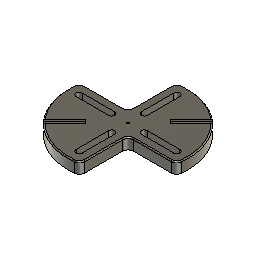
Baseplate (Autodesk Fusion 360 design; units mm, degrees)
part number: 2026-04-13-15-28-07-632
Autodesk Fusion 360 part; units mm, degrees
sketch "Sketch14" plane through (0, 0, 0) normal (0, 0, 1) x (1, 0, 0)
  circle A0 centre (0, 0) radius 55
  dimension "d53" = 110
  constraint coincident A0.centre origin
  measures "d53" diameter of A0
extrude "Extrude9" add sketch "Sketch14" along normal blind 10
sketch "Sketch15" plane through (0, 0, 10) normal (0, 0, 1) x (-1, 0, 0)
  circle A0 centre (0, 0) radius 55
  circle A1 centre (0, 0) radius 15
  circle A2 centre (0, 0) radius 45
  line L0 (-15, 2.8) -> (-45, 2.8)
  arc A3 (-45, 2.8) -> (-45, -2.8) centre (-45, 0) ccw
  line L1 (-45, -2.8) -> (-15, -2.8)
  arc A4 (-15, -2.8) -> (-15, 2.8) centre (-15, 0) ccw
  line L2 (-15, 0) -> (-45, 0) construction
  dimension "d56" = 30
  dimension "d57" = 90
  dimension "d58" = 5.6
  constraint coincident A0.centre A1.centre
  constraint concentric A1 A2
  constraint tangent L0 A3
  constraint tangent A3 L1
  constraint parallel L0 L1
  constraint tangent L1 A4
  constraint tangent L0 A4
  constraint coincident A2 A3.centre
  constraint horizontal L2
  constraint coincident A1 A4.centre
  measures "d56" diameter of A1
  measures "d57" diameter of A2
  measures "d58" diameter of A3
extrude "Extrude10" cut sketch "Sketch15" against normal blind 10 contours A1 A4 | A1 A2 L0 L1 A4 | A2 L0 A3 L1 picked at (-14.0473, 0) picked at (-34.958, -1.556)
pattern_circular "C-Pattern3" count 4 over 360 about axis through (0, 0, 1.75) along (0, 0, 1) of "Extrude10"
sketch "Sketch16" plane through (0, 0, 10) normal (0, 0, 1) x (-1, 0, 0)
  line L0 (2.8, 45) -> (2.8, 15)
  arc A0 (-2.8, 15) -> (2.8, 15) centre (0, 15) ccw
  line L1 (-2.8, 15) -> (-2.8, 45)
  arc A1 (2.8, 45) -> (-2.8, 45) centre (0, 45) ccw
  line L2 (45, -2.8) -> (15, -2.8)
  arc A2 (15, 2.8) -> (15, -2.8) centre (15, 0) ccw
  line L3 (15, 2.8) -> (45, 2.8)
  arc A3 (45, -2.8) -> (45, 2.8) centre (45, 0) ccw
  line L4 (-2.8, -45) -> (-2.8, -15)
  arc A4 (2.8, -15) -> (-2.8, -15) centre (0, -15) ccw
  line L5 (2.8, -15) -> (2.8, -45)
  arc A5 (-2.8, -45) -> (2.8, -45) centre (0, -45) ccw
  line L6 (-45, 2.8) -> (-15, 2.8)
  arc A6 (-15, -2.8) -> (-15, 2.8) centre (-15, 0) ccw
  line L7 (-15, -2.8) -> (-45, -2.8)
  arc A7 (-45, 2.8) -> (-45, -2.8) centre (-45, 0) ccw
  circle A8 centre (0, 0) radius 55
  line L8 (38.3252, 39.4566) -> (-39.4566, -38.3252)
  line L9 (-39.4566, -38.3252) -> (-38.3252, -39.4566)
  line L10 (-38.3252, -39.4566) -> (39.4566, 38.3252)
  line L11 (39.4566, 38.3252) -> (38.3252, 39.4566)
  line L12 (38.3252, 39.4566) -> (-38.3252, -39.4566) construction
  line L13 (-39.4566, -38.3252) -> (39.4566, 38.3252) construction
  line L14 (18.8798, 20.0111) -> (-20.0111, -18.8798)
  line L15 (-20.0111, -18.8798) -> (-18.8798, -20.0111)
  line L16 (-18.8798, -20.0111) -> (20.0111, 18.8798)
  line L17 (20.0111, 18.8798) -> (18.8798, 20.0111)
  line L18 (18.8798, 20.0111) -> (-18.8798, -20.0111) construction
  line L19 (-20.0111, -18.8798) -> (20.0111, 18.8798) construction
  dimension "d63" = 110
  dimension "d64" = 1.6
  dimension "d65" = 55
  dimension "d66" = 1.6
  constraint perpendicular L8 L9
  constraint parallel L8 L10
  constraint parallel L9 L11
  constraint coincident L12 A8.centre
  constraint coincident L13 A8.centre
  constraint coincident A8.centre origin
  constraint perpendicular L14 L15
  constraint parallel L14 L16
  constraint parallel L15 L17
  constraint coincident L18 A8.centre
  constraint coincident L19 A8.centre
  measures "d63" distance of L9.end L10.end
  measures "d64" distance of L8.end L9.end
  measures "d65" distance of L15.end L16.end
  measures "d66" distance of L14.end L15.end
extrude "Extrude11" add sketch "Sketch16" along normal blind 2 contours A8 L8 L10 L17 | A8 L8 L10 L15
sketch "Sketch17" plane through (0, 0, 10) normal (0, 0, 1) x (-1, 0, 0)
  line L0 (18.8798, 20.0111) -> (38.3211, 39.4524)
  arc A0 (38.3211, 39.4524) -> (-39.4524, -38.3211) centre (0, 0) ccw
  line L1 (-39.4524, -38.3211) -> (-20.0111, -18.8798)
  line L2 (-20.0111, -18.8798) -> (-18.8798, -20.0111)
  line L3 (-18.8798, -20.0111) -> (-38.3211, -39.4524)
  arc A1 (-38.3211, -39.4524) -> (39.4524, 38.3211) centre (0, 0) ccw
  line L4 (39.4524, 38.3211) -> (20.0111, 18.8798)
  line L5 (20.0111, 18.8798) -> (18.8798, 20.0111)
  line L6 (2.8, 45) -> (2.8, 15)
  arc A2 (-2.8, 15) -> (2.8, 15) centre (0, 15) ccw
  line L7 (-2.8, 15) -> (-2.8, 45)
  arc A3 (2.8, 45) -> (-2.8, 45) centre (0, 45) ccw
  line L8 (45, -2.8) -> (15, -2.8)
  arc A4 (15, 2.8) -> (15, -2.8) centre (15, 0) ccw
  line L9 (15, 2.8) -> (45, 2.8)
  arc A5 (45, -2.8) -> (45, 2.8) centre (45, 0) ccw
  line L10 (-2.8, -45) -> (-2.8, -15)
  arc A6 (2.8, -15) -> (-2.8, -15) centre (0, -15) ccw
  line L11 (2.8, -15) -> (2.8, -45)
  arc A7 (-2.8, -45) -> (2.8, -45) centre (0, -45) ccw
  line L12 (-45, 2.8) -> (-15, 2.8)
  arc A8 (-15, -2.8) -> (-15, 2.8) centre (-15, 0) ccw
  line L13 (-15, -2.8) -> (-45, -2.8)
  arc A9 (-45, 2.8) -> (-45, -2.8) centre (-45, 0) ccw
  line L14 (-10, 55) -> (10, 55)
  line L15 (10, 55) -> (10, -55)
  line L16 (10, -55) -> (-10, -55)
  line L17 (-10, -55) -> (-10, 55)
  line L18 (-10, 55) -> (10, -55) construction
  line L19 (10, 55) -> (-10, -55) construction
  line L20 (55, 10) -> (-55, 10)
  line L21 (-55, 10) -> (-55, -10)
  line L22 (-55, -10) -> (55, -10)
  line L23 (55, -10) -> (55, 10)
  line L24 (55, 10) -> (-55, -10) construction
  line L25 (-55, 10) -> (55, -10) construction
  dimension "d69" = 110
  dimension "d70" = 110
  dimension "d71" = 20
  constraint horizontal L14
  constraint perpendicular L14 L15
  constraint parallel L14 L16
  constraint parallel L15 L17
  constraint coincident L18 A0.centre
  constraint coincident L19 A0.centre
  constraint coincident A0.centre A1.centre
  constraint horizontal L20
  constraint perpendicular L20 L21
  constraint parallel L20 L22
  constraint parallel L21 L23
  constraint coincident L24 A0.centre
  constraint coincident L25 A0.centre
  measures "d69" distance of L14.end L15.end
  measures "d70" distance of L21.end L22.end
  measures "d71" distance of L20.end L21.end
extrude "Extrude12" cut sketch "Sketch17" against normal blind 10 contours A0 L17 L20 | A1 L15 L22
fillet "Fillet1" radius 5 6 edges at (10, -54.0833, 5) (54.0833, -10, 5) (10, -10, 5) (-54.0833, 10, 5) (-10, 54.0833, 5) (-10, 10, 5)
fillet "Fillet2" radius 1 14 edges at (-18.1001, -51.9364, 10) (8.7081, -53.1035, 10) (10, -32.3747, 10) (11.4645, -11.4645, 10) (32.3747, -10, 10) (53.1035, -8.7081, 10) (51.9364, 18.1001, 10) (-51.9364, -18.1001, 10) (-53.1035, 8.7081, 10) (-32.3747, 10, 10) (-11.4645, 11.4645, 10) (-10, 32.3747, 10) (-8.7081, 53.1035, 10) (18.1001, 51.9364, 10)
sketch "Sketch18" plane through (0, 0, 10) normal (0, 0, 1) x (-1, 0, 0)
  arc A0 (53.7293, -5.4) -> (38.7453, 37.6139) centre (0, 0) ccw
  line L0 (38.7453, 37.6139) -> (20.0111, 18.8798)
  line L1 (20.0111, 18.8798) -> (18.8798, 20.0111)
  line L2 (18.8798, 20.0111) -> (37.6139, 38.7453)
  arc A1 (37.6139, 38.7453) -> (-5.4, 53.7293) centre (0, 0) ccw
  arc A2 (-5.4, 53.7293) -> (-9, 49.7494) centre (-5, 49.7494) ccw
  line L3 (-9, 49.7494) -> (-9, 15)
  arc A3 (-15, 9) -> (-9, 15) centre (-15, 15) ccw
  line L4 (-15, 9) -> (-49.7494, 9)
  arc A4 (-49.7494, 9) -> (-53.7293, 5.4) centre (-49.7494, 5) ccw
  arc A5 (-53.7293, 5.4) -> (-38.7453, -37.6139) centre (0, 0) ccw
  line L5 (-38.7453, -37.6139) -> (-20.0111, -18.8798)
  line L6 (-20.0111, -18.8798) -> (-18.8798, -20.0111)
  line L7 (-18.8798, -20.0111) -> (-37.6139, -38.7453)
  arc A6 (-37.6139, -38.7453) -> (5.4, -53.7293) centre (0, 0) ccw
  arc A7 (5.4, -53.7293) -> (9, -49.7494) centre (5, -49.7494) ccw
  line L8 (9, -49.7494) -> (9, -15)
  arc A8 (15, -9) -> (9, -15) centre (15, -15) ccw
  line L9 (15, -9) -> (49.7494, -9)
  arc A9 (49.7494, -9) -> (53.7293, -5.4) centre (49.7494, -5) ccw
  line L10 (2.8, 45) -> (2.8, 15)
  arc A10 (-2.8, 15) -> (2.8, 15) centre (0, 15) ccw
  line L11 (-2.8, 15) -> (-2.8, 45)
  arc A11 (2.8, 45) -> (-2.8, 45) centre (0, 45) ccw
  line L12 (45, -2.8) -> (15, -2.8)
  arc A12 (15, 2.8) -> (15, -2.8) centre (15, 0) ccw
  line L13 (15, 2.8) -> (45, 2.8)
  arc A13 (45, -2.8) -> (45, 2.8) centre (45, 0) ccw
  line L14 (-2.8, -45) -> (-2.8, -15)
  arc A14 (2.8, -15) -> (-2.8, -15) centre (0, -15) ccw
  line L15 (2.8, -15) -> (2.8, -45)
  arc A15 (-2.8, -45) -> (2.8, -45) centre (0, -45) ccw
  line L16 (-45, 2.8) -> (-15, 2.8)
  arc A16 (-15, -2.8) -> (-15, 2.8) centre (-15, 0) ccw
  line L17 (-15, -2.8) -> (-45, -2.8)
  arc A17 (-45, 2.8) -> (-45, -2.8) centre (-45, 0) ccw
  circle A18 centre (0, 0) radius 1
  dimension "d78" = 2
  constraint coincident A0.centre A1.centre
  measures "d78" diameter of A18
extrude "Extrude13" cut sketch "Sketch18" against normal blind 10 contours A18
